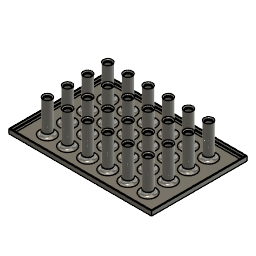
24 deep well led array (Autodesk Fusion 360 design; units mm, degrees)
Autodesk Fusion 360 part; units mm, degrees
sketch "Sketch1" plane through (0, 0, 0) normal (0, 1, 0) x (1, 0, 0)
  line L0 (0, 0) -> (127.5, 0)
  line L1 (127.5, 0) -> (127.5, -85.5)
  line L2 (127.5, -85.5) -> (0, -85.5)
  line L3 (0, -85.5) -> (0, 0)
  line L4 (0, 0) -> (18.75, 0)
  line L5 (18.75, 0) -> (18.75, -15.75)
  line L6 (18.75, -15.75) -> (0, -15.75)
  line L7 (0, -15.75) -> (0, 0)
  line L8 (18.75, -15.75) -> (36.75, -15.75)
  line L9 (36.75, -15.75) -> (36.75, -33.75)
  line L10 (36.75, -33.75) -> (18.75, -33.75)
  line L11 (18.75, -33.75) -> (18.75, -15.75)
  line L12 (36.75, -33.75) -> (54.75, -33.75)
  line L13 (54.75, -33.75) -> (54.75, -51.75)
  line L14 (54.75, -51.75) -> (36.75, -51.75)
  line L15 (36.75, -51.75) -> (36.75, -33.75)
  line L16 (36.75, -51.75) -> (18.75, -51.75)
  line L17 (18.75, -51.75) -> (18.75, -69.75)
  line L18 (18.75, -69.75) -> (36.75, -69.75)
  line L19 (36.75, -69.75) -> (36.75, -51.75)
  line L20 (54.75, -33.75) -> (72.75, -33.75)
  line L21 (72.75, -33.75) -> (72.75, -15.75)
  line L22 (72.75, -15.75) -> (54.75, -15.75)
  line L23 (54.75, -15.75) -> (54.75, -33.75)
  line L24 (54.75, -51.75) -> (72.75, -51.75)
  line L25 (72.75, -51.75) -> (72.75, -69.75)
  line L26 (72.75, -69.75) -> (54.75, -69.75)
  line L27 (54.75, -69.75) -> (54.75, -51.75)
  line L28 (72.75, -51.75) -> (90.75, -51.75)
  line L29 (90.75, -51.75) -> (90.75, -33.75)
  line L30 (90.75, -33.75) -> (72.75, -33.75)
  line L31 (72.75, -33.75) -> (72.75, -51.75)
  line L32 (90.75, -33.75) -> (108.75, -33.75)
  line L33 (108.75, -33.75) -> (108.75, -15.75)
  line L34 (108.75, -15.75) -> (90.75, -15.75)
  line L35 (90.75, -15.75) -> (90.75, -33.75)
  line L36 (90.75, -51.75) -> (108.75, -51.75)
  line L37 (108.75, -51.75) -> (108.75, -69.75)
  line L38 (108.75, -69.75) -> (90.75, -69.75)
  line L39 (90.75, -69.75) -> (90.75, -51.75)
  circle A0 centre (18.75, -69.75) radius 2.75
  circle A1 centre (18.75, -69.75) radius 3
  circle A2 centre (18.75, -69.75) radius 4
  circle A3 centre (36.75, -69.75) radius 2.75
  circle A4 centre (36.75, -69.75) radius 3
  circle A5 centre (36.75, -69.75) radius 4
  circle A6 centre (54.75, -69.75) radius 2.75
  circle A7 centre (54.75, -69.75) radius 3
  circle A8 centre (54.75, -69.75) radius 4
  circle A9 centre (18.75, -51.75) radius 2.75
  circle A10 centre (18.75, -51.75) radius 3
  circle A11 centre (18.75, -51.75) radius 4
  circle A12 centre (36.75, -51.75) radius 2.75
  circle A13 centre (36.75, -51.75) radius 3
  circle A14 centre (36.75, -51.75) radius 4
  circle A15 centre (18.75, -33.75) radius 2.75
  circle A16 centre (18.75, -33.75) radius 3
  circle A17 centre (18.75, -33.75) radius 4
  circle A18 centre (36.75, -33.75) radius 2.75
  circle A19 centre (36.75, -33.75) radius 3
  circle A20 centre (36.75, -33.75) radius 4
  circle A21 centre (54.75, -33.75) radius 2.75
  circle A22 centre (54.75, -33.75) radius 3
  circle A23 centre (54.75, -33.75) radius 4
  circle A24 centre (54.75, -51.75) radius 2.75
  circle A25 centre (54.75, -51.75) radius 3
  circle A26 centre (54.75, -51.75) radius 4
  circle A27 centre (72.75, -69.75) radius 2.75
  circle A28 centre (72.75, -69.75) radius 3
  circle A29 centre (72.75, -69.75) radius 4
  circle A30 centre (72.75, -51.75) radius 2.75
  circle A31 centre (72.75, -51.75) radius 3
  circle A32 centre (72.75, -51.75) radius 4
  circle A33 centre (90.75, -69.75) radius 2.75
  circle A34 centre (90.75, -69.75) radius 3
  circle A35 centre (90.75, -69.75) radius 4
  circle A36 centre (90.75, -51.75) radius 2.75
  circle A37 centre (90.75, -51.75) radius 3
  circle A38 centre (90.75, -51.75) radius 4
  circle A39 centre (108.75, -51.75) radius 2.75
  circle A40 centre (108.75, -51.75) radius 3
  circle A41 centre (108.75, -51.75) radius 4
  circle A42 centre (108.75, -69.75) radius 2.75
  circle A43 centre (108.75, -69.75) radius 3
  circle A44 centre (108.75, -69.75) radius 4
  circle A45 centre (90.75, -33.75) radius 2.75
  circle A46 centre (90.75, -33.75) radius 3
  circle A47 centre (90.75, -33.75) radius 4
  circle A48 centre (72.75, -33.75) radius 2.75
  circle A49 centre (72.75, -33.75) radius 3
  circle A50 centre (72.75, -33.75) radius 4
  circle A51 centre (108.75, -33.75) radius 2.75
  circle A52 centre (108.75, -33.75) radius 3
  circle A53 centre (108.75, -33.75) radius 4
  circle A54 centre (108.75, -15.75) radius 4
  circle A55 centre (90.75, -15.75) radius 4
  circle A56 centre (108.75, -15.75) radius 2.75
  circle A57 centre (108.75, -15.75) radius 3
  circle A58 centre (90.75, -15.75) radius 2.75
  circle A59 centre (90.75, -15.75) radius 3
  circle A60 centre (72.75, -15.75) radius 2.75
  circle A61 centre (72.75, -15.75) radius 3
  circle A62 centre (72.75, -15.75) radius 4
  circle A63 centre (54.75, -15.75) radius 2.75
  circle A64 centre (54.75, -15.75) radius 3
  circle A65 centre (54.75, -15.75) radius 4
  circle A66 centre (36.75, -15.75) radius 2.75
  circle A67 centre (36.75, -15.75) radius 3
  circle A68 centre (36.75, -15.75) radius 4
  circle A69 centre (18.75, -15.75) radius 2.75
  circle A70 centre (18.75, -15.75) radius 3
  circle A71 centre (18.75, -15.75) radius 4
  line L40 (127.5, 0) -> (0, -85.5)
  line L41 (127.5, -85.5) -> (0, 0)
  line L42 (125.75, -83.75) -> (1.75, -83.75)
  line L43 (1.75, -83.75) -> (1.75, -1.75)
  line L44 (1.75, -1.75) -> (125.75, -1.75)
  line L45 (125.75, -1.75) -> (125.75, -83.75)
  line L46 (125.75, -83.75) -> (1.75, -1.75) construction
  line L47 (1.75, -83.75) -> (125.75, -1.75) construction
  point P0 (63.75, -42.75)
  dimension "d1" = 127.5
  dimension "d2" = 85.5
  dimension "d3" = 18.75
  dimension "d4" = 15.75
  dimension "d5" = 18
  dimension "d6" = 18
  dimension "d7" = 18
  dimension "d8" = 18
  dimension "d9" = 18
  dimension "d10" = 18
  dimension "d11" = 18
  dimension "d12" = 18
  dimension "d13" = 18
  dimension "d14" = 18
  dimension "d15" = 18
  dimension "d16" = 18
  dimension "d17" = 18
  dimension "d18" = 18
  dimension "d19" = 18
  dimension "d20" = 18
  dimension "d21" = 5.5
  dimension "d22" = 6
  dimension "d23" = 8
  dimension "d24" = 5.5
  dimension "d25" = 6
  dimension "d26" = 8
  dimension "d27" = 5.5
  dimension "d28" = 6
  dimension "d29" = 8
  dimension "d30" = 5.5
  dimension "d31" = 6
  dimension "d32" = 8
  dimension "d33" = 5.5
  dimension "d34" = 6
  dimension "d35" = 8
  dimension "d36" = 5.5
  dimension "d37" = 6
  dimension "d38" = 8
  dimension "d39" = 5.5
  dimension "d40" = 6
  dimension "d41" = 8
  dimension "d42" = 5.5
  dimension "d43" = 6
  dimension "d44" = 8
  dimension "d45" = 5.5
  dimension "d46" = 6
  dimension "d47" = 8
  dimension "d48" = 5.5
  dimension "d49" = 6
  dimension "d50" = 8
  dimension "d51" = 5.5
  dimension "d52" = 6
  dimension "d53" = 8
  dimension "d54" = 5.5
  dimension "d55" = 6
  dimension "d56" = 8
  dimension "d57" = 5.5
  dimension "d58" = 6
  dimension "d59" = 8
  dimension "d60" = 5.5
  dimension "d61" = 6
  dimension "d62" = 8
  dimension "d63" = 5.5
  dimension "d64" = 6
  dimension "d65" = 8
  dimension "d66" = 5.5
  dimension "d67" = 6
  dimension "d68" = 8
  dimension "d69" = 5.5
  dimension "d70" = 6
  dimension "d71" = 8
  dimension "d72" = 5.5
  dimension "d73" = 6
  dimension "d74" = 8
  dimension "d75" = 8
  dimension "d76" = 8
  dimension "d77" = 5.5
  dimension "d78" = 6
  dimension "d79" = 5.5
  dimension "d80" = 6
  dimension "d81" = 5.5
  dimension "d82" = 6
  dimension "d83" = 8
  dimension "d84" = 5.5
  dimension "d85" = 6
  dimension "d86" = 8
  dimension "d87" = 5.5
  dimension "d88" = 6
  dimension "d89" = 8
  dimension "d90" = 5.5
  dimension "d91" = 6
  dimension "d92" = 8
  dimension "d103" = 124
  dimension "d104" = 82
  constraint horizontal L0
  constraint vertical L1
  constraint horizontal L2
  constraint vertical L3
  constraint coincident L0.start L3.end
  constraint horizontal L4
  constraint vertical L5
  constraint horizontal L6
  constraint vertical L7
  constraint horizontal L8
  constraint vertical L9
  constraint horizontal L10
  constraint vertical L11
  constraint horizontal L12
  constraint vertical L13
  constraint horizontal L14
  constraint vertical L15
  constraint horizontal L16
  constraint vertical L17
  constraint horizontal L18
  constraint vertical L19
  constraint horizontal L20
  constraint vertical L21
  constraint horizontal L22
  constraint vertical L23
  constraint horizontal L24
  constraint vertical L25
  constraint horizontal L26
  constraint vertical L27
  constraint horizontal L28
  constraint vertical L29
  constraint horizontal L30
  constraint vertical L31
  constraint horizontal L32
  constraint vertical L33
  constraint horizontal L34
  constraint vertical L35
  constraint horizontal L36
  constraint vertical L37
  constraint horizontal L38
  constraint vertical L39
  constraint coincident L17.end L18.start
  constraint concentric A0 A2
  constraint coincident L18.end L19.start
  constraint concentric A4 A5
  constraint coincident L26.end L27.start
  constraint concentric A6 A7
  constraint coincident L16.end L17.start
  constraint concentric A9 A10
  constraint concentric A10 A11
  constraint coincident L14.end L15.start
  constraint concentric A12 A13
  constraint concentric A12 A14
  constraint coincident L10.end L11.start
  constraint concentric A15 A16
  constraint concentric A15 A17
  constraint coincident L9.end L10.start
  constraint concentric A18 A19
  constraint concentric A19 A20
  constraint coincident L12.end L13.start
  constraint concentric A21 A23
  constraint coincident L13.end L14.start
  constraint concentric A24 A25
  constraint concentric A25 A26
  constraint coincident L25.end L26.start
  constraint concentric A27 A28
  constraint concentric A28 A29
  constraint coincident L24.end L25.start
  constraint concentric A30 A31
  constraint concentric A31 A32
  constraint coincident L38.end L39.start
  constraint concentric A33 A34
  constraint concentric A34 A35
  constraint coincident L28.end L29.start
  constraint concentric A36 A37
  constraint concentric A37 A38
  constraint coincident L36.end L37.start
  constraint concentric A39 A40
  constraint concentric A39 A41
  constraint coincident L37.end L38.start
  constraint concentric A42 A43
  constraint concentric A42 A44
  constraint coincident L29.end L30.start
  constraint concentric A45 A46
  constraint concentric A45 A47
  constraint coincident L20.end L21.start
  constraint concentric A48 A49
  constraint concentric A49 A50
  constraint coincident L32.end L33.start
  constraint concentric A51 A52
  constraint concentric A52 A53
  constraint coincident L33.end L34.start
  constraint coincident L34.end L35.start
  constraint concentric A54 A56
  constraint concentric A54 A57
  constraint concentric A55 A58
  constraint concentric A58 A59
  constraint coincident L21.end L22.start
  constraint concentric A60 A61
  constraint concentric A60 A62
  constraint coincident L22.end L23.start
  constraint concentric A63 A64
  constraint concentric A63 A65
  constraint coincident L8.end L9.start
  constraint concentric A66 A67
  constraint concentric A67 A68
  constraint coincident L5.end L6.start
  constraint concentric A69 A70
  constraint concentric A70 A71
  constraint horizontal L42
  constraint perpendicular L42 L43
  constraint parallel L42 L44
  constraint parallel L43 L45
  constraint coincident L46 P0
  constraint coincident L47 P0
  constraint midpoint L40 P0
  measures "d1" distance of L0.start L0.end
  measures "d2" distance of L0.start L2.end
  measures "d3" distance of L0.start L4.end
  measures "d4" distance of L0.start L6.end
  measures "d5" distance of L5.end L8.end
  measures "d6" distance of L5.end L10.end
  measures "d7" distance of L9.end L12.end
  measures "d8" distance of L9.end L14.end L12
  measures "d9" distance of L14.end L16.end
  measures "d10" distance of L14.end L18.end
  measures "d11" distance of L12.end L20.end
  measures "d12" distance of L12.end L22.end
  measures "d13" distance of L13.end L24.end
  measures "d14" distance of L13.end L26.end
  measures "d15" distance of L24.end L28.end
  measures "d16" distance of L24.end L20.end
  measures "d17" distance of L29.end L32.end
  measures "d18" distance of L29.end L34.end
  measures "d19" distance of L28.end L36.end
  measures "d20" distance of L28.end L38.end
  measures "d21" diameter of A0
  measures "d22" diameter of A1
  measures "d23" diameter of A2
  measures "d24" diameter of A3
  measures "d25" diameter of A4
  measures "d26" diameter of A5
  measures "d27" diameter of A6
  measures "d28" diameter of A7
  measures "d29" diameter of A8
  measures "d30" diameter of A9
  measures "d31" diameter of A10
  measures "d32" diameter of A11
  measures "d33" diameter of A12
  measures "d34" diameter of A13
  measures "d35" diameter of A14
  measures "d36" diameter of A15
  measures "d37" diameter of A16
  measures "d38" diameter of A17
  measures "d39" diameter of A18
  measures "d40" diameter of A19
  measures "d41" diameter of A20
  measures "d42" diameter of A21
  measures "d43" diameter of A22
  measures "d44" diameter of A23
  measures "d45" diameter of A24
  measures "d46" diameter of A25
  measures "d47" diameter of A26
  measures "d48" diameter of A27
  measures "d49" diameter of A28
  measures "d50" diameter of A29
  measures "d51" diameter of A30
  measures "d52" diameter of A31
  measures "d53" diameter of A32
  measures "d54" diameter of A33
  measures "d55" diameter of A34
  measures "d56" diameter of A35
  measures "d57" diameter of A36
  measures "d58" diameter of A37
  measures "d59" diameter of A38
  measures "d60" diameter of A39
  measures "d61" diameter of A40
  measures "d62" diameter of A41
  measures "d63" diameter of A42
  measures "d64" diameter of A43
  measures "d65" diameter of A44
  measures "d66" diameter of A45
  measures "d67" diameter of A46
  measures "d68" diameter of A47
  measures "d69" diameter of A48
  measures "d70" diameter of A49
  measures "d71" diameter of A50
  measures "d72" diameter of A51
  measures "d73" diameter of A52
  measures "d74" diameter of A53
  measures "d75" diameter of A54
  measures "d76" diameter of A55
  measures "d77" diameter of A56
  measures "d78" diameter of A57
  measures "d79" diameter of A58
  measures "d80" diameter of A59
  measures "d81" diameter of A60
  measures "d82" diameter of A61
  measures "d83" diameter of A62
  measures "d84" diameter of A63
  measures "d85" diameter of A64
  measures "d86" diameter of A65
  measures "d87" diameter of A66
  measures "d88" diameter of A67
  measures "d89" diameter of A68
  measures "d90" diameter of A69
  measures "d91" diameter of A70
  measures "d92" diameter of A71
  measures "d103" distance of L43.end L44.end
  measures "d104" distance of L42.end L43.end
extrude "Extrude1" add sketch "Sketch1" along normal blind 1 contours L3 L6 L7 L41 L43 L44 | L0 L4 L5 L41 L44 | L0 L5 L40 L44 | L3 L6 L40 L42 L43 | L5 A71 L41 L44 | L6 A71 L41 L43 L44 | L1 L40 L41 L42 L44 L45 | L5 L8 L9 L12 L21 L22 L23 L30 L34 L35 A23 A50 A54 A55 A62 A65 A68 A71 L40 L41 L44 | L2 L40 L41 L42 | L6 L10 L11 L15 L16 L17 A2 A11 A14 A17 A20 A71 L40 L42 L43 | L5 L6 A70 A71 L41 | L5 A71 L41 | L29 L32 L33 L36 L37 A38 A41 A44 A47 A53 A54 L40 L41 L42 L44 L45 | L5 A70 A71 L41 | L14 L18 L19 L25 L26 L27 L28 L38 L39 A2 A5 A8 A26 A29 A32 A35 A44 L40 L41 L42 | L6 L11 A70 A71 | L5 A70 L41 | A54 A57 L40 | L33 A54 A57 L40 | L8 A71 L41 | L8 A70 A71 L41 | A1 A2 L40 | L17 A1 A2 L40 | L5 L6 A69 A70 | L6 L11 A69 A70 | L8 L9 L10 L11 A17 A20 A71 L41 | L8 L11 A70 A71 | L5 A69 A70 L41 | A69 A70 L41 | L37 A43 A44 L41 | A43 A44 L41 | L34 A54 A57 L40 | L34 A54 L40 | A56 A57 L40 | L33 A56 A57 L40 | L8 L9 A68 L41 | L8 A69 A70 L41 | L17 L18 A1 A2 | L16 L17 L18 L19 A2 A11 A14 L40 | L18 A1 A2 L40 | L18 A2 L40 | A0 A1 L40 | L17 A0 A1 L40 | L8 L11 A69 A70 | L10 L11 A16 A17 | L10 L11 A16 A17 | L38 A44 L41 | L38 A43 A44 L41 | L37 A42 A43 L41 | A42 A43 L41 | L33 L34 A54 A57 | L32 L33 L34 L35 A47 A53 A54 L40 | L34 A56 A57 L40 | L34 L35 A55 L40 | L8 L9 A67 A68 | L8 L9 A67 A68 | L9 L12 A20 L41 | L16 L17 A10 A11 | L16 L17 A10 A11 | L17 L18 A0 A1 | L18 L19 A5 L40 | L18 A0 A1 L40 | L10 L11 A15 A16 | L10 L11 A15 A16 | L37 L38 A43 A44 | L36 L37 L38 L39 A38 A41 A44 L41 | L38 A42 A43 L41 | L38 L39 A35 L41 | L32 L33 A52 A53 | L32 L33 A52 A53 | L33 L34 A56 A57 | L34 L35 A55 A59 | L34 L35 A55 A59 | L30 L35 A47 L40 | L8 L9 A66 A67 | L8 L9 A66 A67 | L9 L12 A19 A20 | L9 L10 A19 A20 | L12 L13 L14 L15 A14 A20 A23 A26 L40 L41 | L12 A23 L41 | L16 L17 A9 A10 | L16 L17 A9 A10 | L18 L19 A4 A5 | L18 L19 A4 A5 | L14 L19 A14 L40 | L10 L15 A19 A20 | L37 L38 A42 A43 | L38 L39 A34 A35 | L38 L39 A34 A35 | L28 L39 A38 L41 | L36 L37 A40 A41 | L36 L37 A40 A41 | L32 L33 A51 A52 | L32 L33 A51 A52 | L34 L35 A58 A59 | L34 L35 A58 A59 | L32 L35 A46 A47 | L30 L35 A46 A47 | L30 A50 L40 | L28 L29 L30 L31 A32 A38 A47 A50 L40 L41 | L9 L12 A18 A19 | L9 L10 A18 A19 | L12 L15 A19 A20 | L12 L23 A22 A23 | L12 A22 A23 L41 | L13 A22 A23 L41 | L15 L16 A13 A14 | L16 L19 A13 A14 | L18 L19 A3 A4 | L18 L19 A3 A4 | L14 L19 A13 A14 | L14 A26 L40 | L10 L15 A18 A19 | L38 L39 A33 A34 | L38 L39 A33 A34 | L28 L39 A37 A38 | L36 L39 A37 A38 | L28 A32 L41 | L36 L37 A39 A40 | L36 L37 A39 A40 | L29 L32 A46 A47 | L32 L35 A45 A46 | L30 L35 A45 A46 | L29 L30 A46 A47 | L30 A49 A50 L40 | L21 L30 A49 A50 | L31 A49 A50 L40 | L12 L15 A18 A19 | L12 L23 A21 A22 | L12 A21 A22 L41 | L20 L23 A22 A23 | L20 L21 L22 L23 A23 A50 A62 A65 | L13 A23 A26 L40 L41 | L13 A22 A23 L41 | L13 A21 A22 L41 | L15 L16 A12 A13 | L16 L19 A12 A13 | L14 L15 A13 A14 | L14 L19 A12 A13 | L14 A25 A26 L40 | L14 L27 A25 A26 | L13 A25 A26 L40 | L28 L39 A36 A37 | L36 L39 A36 A37 | L28 L29 A37 A38 | L29 L36 A37 A38 | L25 L28 A31 A32 | L28 A31 A32 L41 | L31 A31 A32 L41 | L29 L32 A45 A46 | L29 L30 A45 A46 | L30 A48 A49 L40 | L21 L30 A48 A49 | L20 L21 A49 A50 | L31 A49 A50 L40 | L31 A32 A50 L40 L41 | L31 A48 A49 L40 | L20 L23 A21 A22 | L22 L23 A64 A65 | L22 L23 A64 A65 | L20 A22 A23 L41 | L20 A23 A50 L40 L41 | L13 A22 L41 | L13 A25 A26 L40 | L14 L15 A12 A13 | L14 A24 A25 L40 | L14 L27 A24 A25 | L24 L25 L26 L27 A8 A26 A29 A32 | L24 L27 A25 A26 | L13 A24 A25 L40 | L28 L29 A36 A37 | L29 L36 A36 A37 | L25 L28 A30 A31 | L28 A30 A31 L41 | L24 L25 A31 A32 | L31 A31 A32 L41 | L31 A30 A31 L41 | L20 L21 A48 A49 | L21 L22 A61 A62 | L21 L22 A61 A62 | L20 A49 A50 L40 | L31 A49 L40 | L13 L20 A21 A22 L41 | L22 L23 A63 A64 | L22 L23 A63 A64 | L13 A21 L41 | L13 A25 L40 | L24 A26 A32 L40 L41 | L24 A25 A26 L40 | L24 L27 A24 A25 | L26 L27 A7 A8 | L26 L27 A7 A8 | L24 L25 A30 A31 | L25 L26 A28 A29 | L25 L26 A28 A29 | L24 A31 A32 L41 | L31 A31 L41 | L20 L31 A48 A49 L40 | L21 L22 A60 A61 | L21 L22 A60 A61 | L31 A48 L40 | L13 L24 A24 A25 L40 | L13 A24 L40 | L26 L27 A6 A7 | L26 L27 A6 A7 | L24 L31 A30 A31 L41 | L25 L26 A27 A28 | L25 L26 A27 A28 | L31 A30 L41
extrude "Extrude2" add sketch "Sketch1" along normal blind 30 contours L5 L6 A70 A71 L41 | L5 A71 L41 | L5 A70 A71 L41 | L6 L11 A70 A71 | L5 A70 L41 | A54 A57 L40 | L33 A54 A57 L40 | L8 A70 A71 L41 | A1 A2 L40 | L17 A1 A2 L40 | L8 L11 A70 A71 | L37 A43 A44 L41 | A43 A44 L41 | L34 A54 A57 L40 | L17 L18 A1 A2 | L18 A1 A2 L40 | L10 L11 A16 A17 | L10 L11 A16 A17 | L38 A43 A44 L41 | L33 L34 A54 A57 | L8 L9 A67 A68 | L8 L9 A67 A68 | L16 L17 A10 A11 | L16 L17 A10 A11 | L37 L38 A43 A44 | L32 L33 A52 A53 | L32 L33 A52 A53 | L34 L35 A55 A59 | L34 L35 A55 A59 | L9 L12 A19 A20 | L9 L10 A19 A20 | L18 L19 A4 A5 | L18 L19 A4 A5 | L10 L15 A19 A20 | L38 L39 A34 A35 | L38 L39 A34 A35 | L36 L37 A40 A41 | L36 L37 A40 A41 | L32 L35 A46 A47 | L30 L35 A46 A47 | L12 L15 A19 A20 | L12 L23 A22 A23 | L12 A22 A23 L41 | L13 A22 A23 L41 | L15 L16 A13 A14 | L16 L19 A13 A14 | L14 L19 A13 A14 | L28 L39 A37 A38 | L36 L39 A37 A38 | L29 L32 A46 A47 | L29 L30 A46 A47 | L30 A49 A50 L40 | L21 L30 A49 A50 | L31 A49 A50 L40 | L20 L23 A22 A23 | L13 A22 A23 L41 | L14 L15 A13 A14 | L14 A25 A26 L40 | L14 L27 A25 A26 | L13 A25 A26 L40 | L28 L29 A37 A38 | L29 L36 A37 A38 | L25 L28 A31 A32 | L28 A31 A32 L41 | L31 A31 A32 L41 | L20 L21 A49 A50 | L31 A49 A50 L40 | L22 L23 A64 A65 | L22 L23 A64 A65 | L20 A22 A23 L41 | L13 A25 A26 L40 | L24 L27 A25 A26 | L24 L25 A31 A32 | L31 A31 A32 L41 | L21 L22 A61 A62 | L21 L22 A61 A62 | L20 A49 A50 L40 | L24 A25 A26 L40 | L26 L27 A7 A8 | L26 L27 A7 A8 | L25 L26 A28 A29 | L25 L26 A28 A29 | L24 A31 A32 L41
extrude "Extrude3" add 24 faces at (21.6453, 1, 15.4643) (39.6453, 1, 15.4643) (51.8992, 1, 16.3304) (70.4333, 1, 17.5099) (111.6008, 1, 16.3304) (93.6453, 1, 15.4643) (88.4333, 1, 35.5099) (105.8547, 1, 33.4643) (75.5703, 1, 33.036) (57.5703, 1, 33.036) (39.2346, 1, 32.2364) (19.2512, 1, 36.6158) (19.2512, 1, 54.6158) (39.2346, 1, 50.2364) (53.055, 1, 54.1145) (69.8547, 1, 51.4643) (87.8547, 1, 51.4643) (111.4825, 1, 52.7488) (111.0667, 1, 71.5099) (89.8272, 1, 72.5091) (18.3842, 1, 66.8638) (39.4324, 1, 68.6236) (54.8185, 1, 72.6585) (69.8992, 1, 70.3304) along direction (0, 1, 0) blind 27
extrude "Extrude4" add sketch "Sketch1" along normal blind 4 contours L3 L6 L7 L41 L43 L44 | L0 L4 L5 L41 L44 | L0 L5 L40 L44 | L3 L6 L40 L42 L43 | L1 L40 L41 L42 L44 L45 | L2 L40 L41 L42
fillet "Fillet1" radius 3 24 edges at (105.0207, 1, 68.3035) (105.0207, 1, 50.3035) (87.0207, 1, 68.3035) (87.0207, 1, 50.3035) (105.0207, 1, 32.3035) (87.0207, 1, 32.3035) (69.0207, 1, 32.3035) (69.0207, 1, 50.3035) (51.0207, 1, 50.3035) (69.0207, 1, 68.3035) (51.0207, 1, 68.3035) (33.0207, 1, 68.3035) (33.0207, 1, 50.3035) (15.0207, 1, 50.3035) (15.0207, 1, 68.3035) (15.0207, 1, 32.3035) (33.0207, 1, 32.3035) (51.0207, 1, 32.3035) (105.0207, 1, 14.3035) (87.0207, 1, 14.3035) (69.0207, 1, 14.3035) (51.0207, 1, 14.3035) (33.0207, 1, 14.3035) (15.0207, 1, 14.3035)
fillet "Fillet2" radius 1 32 edges at (15.953, 30, 14.6652) (33.953, 30, 14.6652) (51.953, 30, 14.6652) (69.953, 30, 14.6652) (87.953, 30, 14.6652) (87.953, 30, 32.6652) (69.953, 30, 32.6652) (51.953, 30, 32.6652) (33.953, 30, 32.6652) (15.953, 30, 32.6652) (15.953, 30, 50.6652) (15.953, 30, 68.6652) (33.953, 30, 68.6652) (33.953, 30, 50.6652) (51.953, 30, 50.6652) (51.953, 30, 68.6652) (69.953, 30, 68.6652) (69.953, 30, 50.6652) (87.953, 30, 50.6652) (87.953, 30, 68.6652) (105.953, 30, 68.6652) (105.953, 30, 50.6652) (105.953, 30, 32.6652) (105.953, 30, 14.6652) (63.75, 4, 1.75) (125.75, 4, 42.75) (1.75, 4, 42.75) (63.75, 4, 83.75) (1.75, 1, 42.75) (63.75, 1, 1.75) (125.75, 1, 42.75) (63.75, 1, 83.75)
